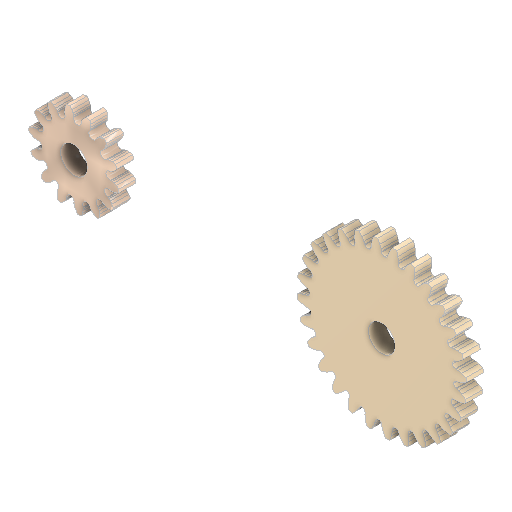
# Autodesk Inventor part: tool_kit
Saved by Autodesk Inventor 2025.3 (Build 293356030, 356C)
## iProperties
Created: 2025-09-03
Part Number: tool_kit
Material: 一般
Document SubType Name: Modeling
Designer: 陳泓任
Density: 1 g/cm^3
Appearance: 一般
Author: 陳泓任
Autodesk Inventor part; units mm, degrees
(part 1 of 2)
ref_plane "YZ Plane" through (0, 0, 0) normal (1, 0, 0) x (0, 1, 0)
ref_plane "XZ Plane" through (0, 0, 0) normal (0, 1, 0) x (-1, 0, 0)
ref_plane "XY Plane" through (0, 0, 0) normal (0, 0, 1) x (1, 0, 0)
sketch "草圖2" plane through (0, 0, 0) normal (0, 0, 1) x (1, 0, 0)
  circle A0 centre (1.2232, 0.0647) radius 2.34
  arc A1 (5.8477, -6.4632) -> (5.8053, -5.9159) centre (1.4586, -6.5279) ccw
  arc A2 (5.8053, -5.9159) -> (5.7115, -5.4774) centre (2.6173, -6.3691) ccw
  arc A3 (5.7115, -5.4774) -> (5.6019, -5.1764) centre (3.4971, -6.1133) ccw
  arc A4 (5.6019, -5.1764) -> (5.5121, -5.0064) centre (4.3299, -5.7392) ccw
  arc A5 (5.5121, -5.0064) -> (5.4754, -4.9539) centre (5.071, -5.2755) ccw
  line L0 (5.4754, -4.9539) -> (5.4708, -4.9484)
  arc A6 (6.3664, -4.0369) -> (5.4708, -4.9484) centre (5.8051, -4.3811) ccw
  arc A7 (6.3664, -4.0369) -> (6.4195, -4.0716) centre (6.6754, -3.6228) ccw
  arc A8 (6.4195, -4.0716) -> (6.5921, -4.1563) centre (7.1169, -2.8681) ccw
  arc A9 (6.5921, -4.1563) -> (6.8962, -4.2569) centre (7.466, -2.0246) ccw
  arc A10 (6.8962, -4.2569) -> (7.3374, -4.3377) centre (7.6956, -1.1376) ccw
  arc A11 (7.3374, -4.3377) -> (7.8856, -4.3638) centre (7.8199, 0.0253) ccw
  arc A12 (8.2221, -3.8102) -> (7.9465, -3.3355) centre (4.2957, -5.7729) ccw
  arc A13 (7.9465, -3.3355) -> (7.6716, -2.9812) centre (5.2708, -5.1271) ccw
  arc A14 (7.6716, -2.9812) -> (7.4423, -2.7575) centre (5.9524, -4.5148) ccw
  arc A15 (7.4423, -2.7575) -> (7.2877, -2.6433) centre (6.5404, -3.8165) ccw
  arc A16 (7.2877, -2.6433) -> (7.2318, -2.6119) centre (7.007, -3.0771) ccw
  line L1 (7.2318, -2.6119) -> (7.2252, -2.609)
  arc A17 (7.6367, -1.3991) -> (7.2252, -2.609) centre (7.2803, -1.9528) ccw
  arc A18 (7.6367, -1.3991) -> (7.6996, -1.4074) centre (7.7354, -0.8919) ccw
  arc A19 (7.6996, -1.4074) -> (7.8918, -1.4088) centre (7.8057, -0.0205) ccw
  arc A20 (7.8918, -1.4088) -> (8.2095, -1.3675) centre (7.7543, 0.891) ccw
  arc A21 (8.2095, -1.3675) -> (8.642, -1.2489) centre (7.5763, 1.7897) ccw
  arc A22 (8.642, -1.2489) -> (9.1473, -1.0345) centre (7.1837, 2.8914) ccw
  arc A23 (9.2102, -0.3897) -> (8.756, -0.0817) centre (6.5243, -3.8616) ccw
  arc A24 (8.756, -0.0817) -> (8.3546, 0.1183) centre (7.1226, -2.8567) ccw
  arc A25 (8.3546, 0.1183) -> (8.0509, 0.2203) centre (7.4711, -2.0094) ccw
  arc A26 (8.0509, 0.2203) -> (7.8621, 0.2562) centre (7.6979, -1.1251) ccw
  arc A27 (7.8621, 0.2562) -> (7.7981, 0.2602) centre (7.7974, -0.2565) ccw
  line L2 (7.7981, 0.2602) -> (7.7909, 0.26)
  arc A28 (7.6367, 1.5286) -> (7.7909, 0.26) centre (7.5559, 0.8751) ccw
  arc A29 (7.6367, 1.5286) -> (7.697, 1.5484) centre (7.5055, 2.0283) ccw
  arc A30 (7.697, 1.5484) -> (7.8707, 1.6306) centre (7.1908, 2.844) ccw
  arc A31 (7.8707, 1.6306) -> (8.139, 1.8056) centre (6.749, 3.6429) ccw
  arc A32 (8.139, 1.8056) -> (8.4772, 2.1001) centre (6.1987, 4.3754) ccw
  arc A33 (8.4772, 2.1001) -> (8.8395, 2.5125) centre (5.3669, 5.1976) ccw
  arc A34 (8.6164, 3.1207) -> (8.0735, 3.2012) centre (7.7029, -1.1727) ccw
  arc A35 (8.0735, 3.2012) -> (7.6251, 3.2072) centre (7.8059, -0.0077) ccw
  arc A36 (7.6251, 3.2072) -> (7.3072, 3.1674) centre (7.7522, 0.9069) ccw
  arc A37 (7.3072, 3.1674) -> (7.1215, 3.1177) centre (7.5729, 1.802) ccw
  arc A38 (7.1215, 3.1177) -> (7.0622, 3.0936) centre (7.2857, 2.6278) ccw
  line L3 (7.0622, 3.0936) -> (7.0558, 3.0903)
  arc A39 (6.3664, 4.1663) -> (7.0558, 3.0903) centre (6.5771, 3.5425) ccw
  arc A40 (6.3664, 4.1663) -> (6.4121, 4.2104) centre (6.0314, 4.5597) ccw
  arc A41 (6.4121, 4.2104) -> (6.533, 4.3598) centre (5.3939, 5.158) ccw
  arc A42 (6.533, 4.3598) -> (6.6988, 4.6339) centre (4.6492, 5.6861) ccw
  arc A43 (6.6988, 4.6339) -> (6.8757, 5.046) centre (3.8356, 6.1073) ccw
  arc A44 (6.8757, 5.046) -> (7.0232, 5.5747) centre (2.7295, 6.4872) ccw
  arc A45 (6.5583, 6.0259) -> (6.0342, 5.8628) centre (7.5981, 1.7613) ccw
  arc A46 (6.0342, 5.8628) -> (5.6276, 5.6737) centre (7.1855, 2.8556) ccw
  arc A47 (5.6276, 5.6737) -> (5.3585, 5.4999) centre (6.7402, 3.6563) ccw
  arc A48 (5.3585, 5.4999) -> (5.2128, 5.3746) centre (6.1903, 4.385) ccw
  arc A49 (5.2128, 5.3746) -> (5.1697, 5.3271) centre (5.5733, 5.0044) ccw
  line L4 (5.1697, 5.3271) -> (5.1654, 5.3214)
  arc A50 (4.0774, 5.9917) -> (5.1654, 5.3214) centre (4.538, 5.5211) ccw
  arc A51 (4.0774, 5.9917) -> (4.0995, 6.0512) centre (3.6049, 6.2008) ccw
  arc A52 (4.0995, 6.0512) -> (4.1436, 6.2383) centre (2.771, 6.4633) ccw
  arc A53 (4.1436, 6.2383) -> (4.174, 6.5572) centre (1.8709, 6.6159) ccw
  arc A54 (4.174, 6.5572) -> (4.1547, 7.0052) centre (0.9551, 6.6424) ccw
  arc A55 (4.1547, 7.0052) -> (4.0581, 7.5456) centre (-0.2063, 6.5048) ccw
  arc A56 (3.4435, 7.7504) -> (3.0421, 7.3761) centre (6.2307, 4.3592) ccw
  arc A57 (3.0421, 7.3761) -> (2.7578, 7.0293) centre (5.3841, 5.1662) ccw
  arc A58 (2.7578, 7.0293) -> (2.5908, 6.7559) centre (4.6355, 5.6944) ccw
  arc A59 (2.5908, 6.7559) -> (2.5138, 6.5798) centre (3.8239, 6.1123) ccw
  arc A60 (2.5138, 6.5798) -> (2.4956, 6.5183) centre (2.9992, 6.4027) ccw
  line L5 (2.4956, 6.5183) -> (2.4942, 6.5113)
  arc A61 (1.2231, 6.6432) -> (2.4942, 6.5113) centre (1.8423, 6.419) ccw
  arc A62 (1.2231, 6.6432) -> (1.2172, 6.7064) centre (0.7067, 6.6265) ccw
  arc A63 (1.2172, 6.7064) -> (1.1758, 6.8941) centre (-0.1585, 6.5012) ccw
  arc A64 (1.1758, 6.8941) -> (1.0648, 7.1946) centre (-1.0357, 6.2482) ccw
  arc A65 (1.0648, 7.1946) -> (0.853, 7.5898) centre (-1.8723, 5.8747) ccw
  arc A66 (0.853, 7.5898) -> (0.5315, 8.0348) centre (-2.859, 5.2468) ccw
  arc A67 (-0.1111, 7.9527) -> (-0.3103, 7.4412) centre (3.8715, 6.1066) ccw
  arc A68 (-0.3103, 7.4412) -> (-0.416, 7.0054) centre (2.7586, 6.4663) ccw
  arc A69 (-0.416, 7.0054) -> (-0.4479, 6.6866) centre (1.855, 6.6175) ccw
  arc A70 (-0.4479, 6.6866) -> (-0.4408, 6.4946) centre (0.9423, 6.6418) ccw
  arc A71 (-0.4408, 6.4946) -> (-0.4305, 6.4313) centre (0.0734, 6.5456) ccw
  line L6 (-0.4305, 6.4313) -> (-0.4287, 6.4244)
  arc A72 (-1.6311, 5.9917) -> (-0.4287, 6.4244) centre (-0.9761, 6.0583) ccw
  arc A73 (-1.6311, 5.9917) -> (-1.6639, 6.0461) centre (-2.0892, 5.7526) ccw
  arc A74 (-1.6639, 6.0461) -> (-1.7775, 6.1914) centre (-2.8144, 5.2643) ccw
  arc A75 (-1.7775, 6.1914) -> (-2.013, 6.4198) centre (-3.4949, 4.6558) ccw
  arc A76 (-2.013, 6.4198) -> (-2.3754, 6.684) centre (-4.0866, 3.9563) ccw
  arc A77 (-2.3754, 6.684) -> (-2.858, 6.9454) centre (-4.7032, 2.9624) ccw
  arc A78 (-3.4014, 6.5926) -> (-3.359, 6.0454) centre (0.9877, 6.6573) ccw
  arc A79 (-3.359, 6.0454) -> (-3.2651, 5.6068) centre (-0.171, 6.4986) ccw
  arc A80 (-3.2651, 5.6068) -> (-3.1555, 5.3058) centre (-1.0507, 6.2427) ccw
  arc A81 (-3.1555, 5.3058) -> (-3.0658, 5.1359) centre (-1.8836, 5.8686) ccw
  arc A82 (-3.0658, 5.1359) -> (-3.0291, 5.0833) centre (-2.6247, 5.4049) ccw
  line L7 (-3.0291, 5.0833) -> (-3.0245, 5.0778)
  arc A83 (-3.9201, 4.1663) -> (-3.0245, 5.0778) centre (-3.3588, 4.5106) ccw
  arc A84 (-3.9201, 4.1663) -> (-3.9732, 4.2011) centre (-4.2291, 3.7522) ccw
  arc A85 (-3.9732, 4.2011) -> (-4.1458, 4.2857) centre (-4.6705, 2.9976) ccw
  arc A86 (-4.1458, 4.2857) -> (-4.4499, 4.3863) centre (-5.0197, 2.154) ccw
  arc A87 (-4.4499, 4.3863) -> (-4.891, 4.4671) centre (-5.2493, 1.2671) ccw
  arc A88 (-4.891, 4.4671) -> (-5.4393, 4.4932) centre (-5.3735, 0.1041) ccw
  arc A89 (-5.7758, 3.9396) -> (-5.5002, 3.465) centre (-1.8494, 5.9023) ccw
  arc A90 (-5.5002, 3.465) -> (-5.2253, 3.1106) centre (-2.8245, 5.2565) ccw
  arc A91 (-5.2253, 3.1106) -> (-4.9959, 2.887) centre (-3.5061, 4.6443) ccw
  arc A92 (-4.9959, 2.887) -> (-4.8413, 2.7727) centre (-4.0941, 3.9459) ccw
  arc A93 (-4.8413, 2.7727) -> (-4.7855, 2.7413) centre (-4.5607, 3.2066) ccw
  line L8 (-4.7855, 2.7413) -> (-4.7789, 2.7384)
  arc A94 (-5.1904, 1.5285) -> (-4.7789, 2.7384) centre (-4.834, 2.0823) ccw
  arc A95 (-5.1904, 1.5285) -> (-5.2533, 1.5368) centre (-5.2891, 1.0214) ccw
  arc A96 (-5.2533, 1.5368) -> (-5.4455, 1.5382) centre (-5.3594, 0.1499) ccw
  arc A97 (-5.4455, 1.5382) -> (-5.7632, 1.4969) centre (-5.3079, -0.7616) ccw
  arc A98 (-5.7632, 1.4969) -> (-6.1957, 1.3783) centre (-5.13, -1.6603) ccw
  arc A99 (-6.1957, 1.3783) -> (-6.701, 1.1639) centre (-4.7374, -2.762) ccw
  arc A100 (-6.7522, 0.6928) -> (-6.7639, 0.5192) centre (1.2232, 0.0647) ccw
  arc A101 (-6.7639, 0.5192) -> (-6.3096, 0.2111) centre (-4.078, 3.9911) ccw
  arc A102 (-6.3096, 0.2111) -> (-5.9009, 0.0081) centre (-4.6763, 2.9861) ccw
  arc A103 (-5.9009, 0.0081) -> (-5.6046, -0.0909) centre (-5.0247, 2.1388) ccw
  arc A104 (-5.6046, -0.0909) -> (-5.4157, -0.1267) centre (-5.2515, 1.2545) ccw
  arc A105 (-5.4157, -0.1267) -> (-5.3518, -0.1308) centre (-5.3511, 0.3859) ccw
  line L9 (-5.3518, -0.1308) -> (-5.3446, -0.1306)
  arc A106 (-5.1903, -1.3991) -> (-5.3446, -0.1306) centre (-5.1095, -0.7457) ccw
  arc A107 (-5.1903, -1.3991) -> (-5.2506, -1.419) centre (-5.0592, -1.8989) ccw
  arc A108 (-5.2506, -1.419) -> (-5.4244, -1.5011) centre (-4.7445, -2.7146) ccw
  arc A109 (-5.4244, -1.5011) -> (-5.6927, -1.6762) centre (-4.3027, -3.5135) ccw
  arc A110 (-5.6927, -1.6762) -> (-6.0309, -1.9707) centre (-3.7524, -4.246) ccw
  arc A111 (-6.0309, -1.9707) -> (-6.3932, -2.3831) centre (-2.9206, -5.0682) ccw
  arc A112 (-6.1701, -2.9913) -> (-5.6272, -3.0718) centre (-5.2566, 1.3022) ccw
  arc A113 (-5.6272, -3.0718) -> (-5.1787, -3.0778) centre (-5.3596, 0.1372) ccw
  arc A114 (-5.1787, -3.0778) -> (-4.8609, -3.0379) centre (-5.3059, -0.7775) ccw
  arc A115 (-4.8609, -3.0379) -> (-4.6752, -2.9883) centre (-5.1266, -1.6726) ccw
  arc A116 (-4.6752, -2.9883) -> (-4.6158, -2.9642) centre (-4.8394, -2.4984) ccw
  line L10 (-4.6158, -2.9642) -> (-4.6095, -2.9609)
  arc A117 (-3.9201, -4.0369) -> (-4.6095, -2.9609) centre (-4.1308, -3.4131) ccw
  arc A118 (-3.9201, -4.0369) -> (-3.9658, -4.0809) centre (-3.5851, -4.4303) ccw
  arc A119 (-3.9658, -4.0809) -> (-4.0867, -4.2304) centre (-2.9476, -5.0286) ccw
  arc A120 (-4.0867, -4.2304) -> (-4.2488, -4.4974) centre (-2.2029, -5.5567) ccw
  arc A121 (-4.2488, -4.4974) -> (-4.4294, -4.9166) centre (-1.3893, -5.9779) ccw
  arc A122 (-4.4294, -4.9166) -> (-4.5769, -5.4453) centre (-0.2832, -6.3578) ccw
  arc A123 (-4.112, -5.8965) -> (-3.5879, -5.7334) centre (-5.1518, -1.6318) ccw
  arc A124 (-3.5879, -5.7334) -> (-3.1813, -5.5443) centre (-4.7392, -2.7262) ccw
  arc A125 (-3.1813, -5.5443) -> (-2.9122, -5.3705) centre (-4.2939, -3.5269) ccw
  arc A126 (-2.9122, -5.3705) -> (-2.7665, -5.2451) centre (-3.7439, -4.2556) ccw
  arc A127 (-2.7665, -5.2451) -> (-2.7234, -5.1977) centre (-3.1269, -4.875) ccw
  line L11 (-2.7234, -5.1977) -> (-2.7191, -5.1919)
  arc A128 (-1.6311, -5.8623) -> (-2.7191, -5.1919) centre (-2.0916, -5.3917) ccw
  arc A129 (-1.6311, -5.8623) -> (-1.6532, -5.9218) centre (-1.1586, -6.0713) ccw
  arc A130 (-1.6532, -5.9218) -> (-1.6973, -6.1089) centre (-0.3247, -6.3338) ccw
  arc A131 (-1.6973, -6.1089) -> (-1.7277, -6.4278) centre (0.5754, -6.4865) ccw
  arc A132 (-1.7277, -6.4278) -> (-1.7083, -6.8758) centre (1.4912, -6.513) ccw
  arc A133 (-1.7083, -6.8758) -> (-1.6118, -7.4161) centre (2.6526, -6.3754) ccw
  arc A134 (-0.9972, -7.621) -> (-0.5958, -7.2467) centre (-3.7844, -4.2298) ccw
  arc A135 (-0.5958, -7.2467) -> (-0.3114, -6.8998) centre (-2.9378, -5.0367) ccw
  arc A136 (-0.3114, -6.8998) -> (-0.1444, -6.6265) centre (-2.1892, -5.565) ccw
  arc A137 (-0.1444, -6.6265) -> (-0.0675, -6.4503) centre (-1.3775, -5.9829) ccw
  arc A138 (-0.0675, -6.4503) -> (-0.0493, -6.3889) centre (-0.5529, -6.2733) ccw
  line L12 (-0.0493, -6.3889) -> (-0.0479, -6.3818)
  arc A139 (1.2232, -6.5137) -> (-0.0479, -6.3818) centre (0.604, -6.2895) ccw
  arc A140 (1.2232, -6.5137) -> (1.2291, -6.5769) centre (1.7396, -6.4971) ccw
  arc A141 (1.2291, -6.5769) -> (1.2705, -6.7646) centre (2.6048, -6.3718) ccw
  arc A142 (1.2705, -6.7646) -> (1.3815, -7.0651) centre (3.482, -6.1188) ccw
  arc A143 (1.3815, -7.0651) -> (1.5934, -7.4604) centre (4.3186, -5.7453) ccw
  arc A144 (1.5934, -7.4604) -> (1.9148, -7.9053) centre (5.3053, -5.1174) ccw
  arc A145 (2.5574, -7.8232) -> (2.7567, -7.3118) centre (-1.4251, -5.9772) ccw
  arc A146 (2.7567, -7.3118) -> (2.8623, -6.876) centre (-0.3123, -6.3369) ccw
  arc A147 (2.8623, -6.876) -> (2.8944, -6.5495) centre (0.5914, -6.4881) ccw
  arc A148 (2.8944, -6.5495) -> (2.8871, -6.3651) centre (1.504, -6.5124) ccw
  arc A149 (2.8871, -6.3651) -> (2.8768, -6.3019) centre (2.3729, -6.4162) ccw
  line L13 (2.8768, -6.3019) -> (2.875, -6.2949)
  arc A150 (4.0775, -5.8623) -> (2.875, -6.2949) centre (3.4224, -5.9289) ccw
  arc A151 (4.0775, -5.8623) -> (4.1102, -5.9166) centre (4.5355, -5.6232) ccw
  arc A152 (4.1102, -5.9166) -> (4.2238, -6.062) centre (5.2607, -5.1349) ccw
  arc A153 (4.2238, -6.062) -> (4.4593, -6.2904) centre (5.9412, -4.5263) ccw
  arc A154 (4.4593, -6.2904) -> (4.8217, -6.5546) centre (6.533, -3.8269) ccw
  arc A155 (4.8217, -6.5546) -> (5.3044, -6.816) centre (7.1495, -2.833) ccw
  circle A156 centre (55.7173, -0.0187) radius 2.34
  arc A157 (58.5817, 13.954) -> (58.37, 14.7449) centre (52.2673, 12.6876) ccw
  arc A158 (58.6643, 13.3186) -> (58.5817, 13.954) centre (54.0648, 13.0435) ccw
  arc A159 (58.6615, 12.9342) -> (58.6643, 13.3186) centre (55.8878, 13.1464) ccw
  arc A160 (58.6513, 12.844) -> (58.6615, 12.9342) centre (57.6307, 13.0057) ccw
  arc A161 (58.6513, 12.844) -> (59.051, 12.288) centre (59.177, 12.8002) ccw
  line L14 (59.051, 12.288) -> (59.0514, 12.2894)
  arc A162 (59.0514, 12.2894) -> (59.0647, 12.2848) centre (59.2291, 12.7861) ccw
  arc A163 (59.0647, 12.2848) -> (59.0785, 12.282) centre (59.177, 12.8002) ccw
  line L15 (59.0785, 12.282) -> (59.0782, 12.2806)
  arc A164 (59.0782, 12.2806) -> (59.7045, 12.5575) centre (59.2291, 12.7861) ccw
  arc A165 (59.7413, 12.6404) -> (59.7045, 12.5575) centre (60.6663, 12.1798) ccw
  arc A166 (59.9337, 12.9733) -> (59.7413, 12.6404) centre (62.2403, 11.4181) ccw
  arc A167 (60.3268, 13.4792) -> (59.9337, 12.9733) centre (63.7598, 10.4058) ccw
  arc A168 (60.91, 14.0538) -> (60.3268, 13.4792) centre (65.1293, 9.1883) ccw
  arc A169 (61.6191, 12.9663) -> (61.5887, 13.7845) centre (55.1812, 13.1367) ccw
  arc A170 (61.5583, 12.3285) -> (61.6191, 12.9663) centre (57.0128, 13.0837) ccw
  arc A171 (61.47, 11.9543) -> (61.5583, 12.3285) centre (58.813, 12.7784) ccw
  arc A172 (61.44, 11.8687) -> (61.47, 11.9543) centre (60.4809, 12.2534) ccw
  arc A173 (61.44, 11.8687) -> (61.7059, 11.2376) centre (61.9427, 11.709) ccw
  line L16 (61.7059, 11.2376) -> (61.7066, 11.2389)
  arc A174 (61.7066, 11.2389) -> (61.7186, 11.2315) centre (61.9903, 11.6836) ccw
  arc A175 (61.7186, 11.2315) -> (61.7314, 11.2257) centre (61.9427, 11.709) ccw
  line L17 (61.7314, 11.2257) -> (61.7308, 11.2244)
  arc A176 (61.7308, 11.2244) -> (62.403, 11.355) centre (61.9903, 11.6836) ccw
  arc A177 (62.4574, 11.4276) -> (62.403, 11.355) centre (63.2567, 10.7727) ccw
  arc A178 (62.719, 11.7093) -> (62.4574, 11.4276) centre (64.6216, 9.6799) ccw
  arc A179 (63.2148, 12.115) -> (62.719, 11.7093) centre (65.8779, 8.3548) ccw
  arc A180 (63.9113, 12.5455) -> (63.2148, 12.115) centre (66.942, 6.8631) ccw
  arc A181 (64.3605, 11.3274) -> (64.513, 12.1319) centre (58.122, 12.9262) ccw
  arc A182 (64.1593, 10.7192) -> (64.3605, 11.3274) centre (59.8959, 12.467) ccw
  arc A183 (63.99, 10.374) -> (64.1593, 10.7192) centre (61.583, 11.7687) ccw
  arc A184 (63.9417, 10.2972) -> (63.99, 10.374) centre (63.0923, 10.8857) ccw
  arc A185 (63.9417, 10.2972) -> (64.0605, 9.6228) centre (64.3963, 10.0297) ccw
  line L18 (64.0605, 9.6228) -> (64.0615, 9.6239)
  arc A186 (64.0615, 9.6239) -> (64.0715, 9.614) centre (64.4371, 9.9943) ccw
  arc A187 (64.0715, 9.614) -> (64.0828, 9.6055) centre (64.3963, 10.0297) ccw
  line L19 (64.0828, 9.6055) -> (64.0818, 9.6044)
  arc A188 (64.0818, 9.6044) -> (64.7662, 9.5821) centre (64.4371, 9.9943) ccw
  arc A189 (64.8354, 9.6409) -> (64.7662, 9.5821) centre (65.469, 8.8245) ccw
  arc A190 (65.1531, 9.8572) -> (64.8354, 9.6409) centre (66.5565, 7.4553) ccw
  arc A191 (65.7268, 10.1425) -> (65.1531, 9.8572) centre (67.4864, 5.8839) ccw
  arc A192 (66.5016, 10.4072) -> (65.7268, 10.1425) centre (68.1919, 4.1928) ccw
  arc A193 (66.6686, 9.1197) -> (66.9962, 9.87) centre (60.9422, 12.0665) ccw
  arc A194 (66.3371, 8.5714) -> (66.6686, 9.1197) centre (62.5695, 11.2241) ccw
  arc A195 (66.0952, 8.2726) -> (66.3371, 8.5714) centre (64.0589, 10.1679) ccw
  arc A196 (66.031, 8.2085) -> (66.0952, 8.2726) centre (65.3338, 8.9713) ccw
  arc A197 (66.031, 8.2085) -> (65.9968, 7.5246) centre (66.4147, 7.8465) ccw
  line L20 (65.9968, 7.5246) -> (65.998, 7.5254)
  arc A198 (65.998, 7.5254) -> (66.0055, 7.5135) centre (66.4466, 7.8029) ccw
  arc A199 (66.0055, 7.5135) -> (66.0146, 7.5027) centre (66.4147, 7.8465) ccw
  line L21 (66.0146, 7.5027) -> (66.0134, 7.5018)
  arc A200 (66.0134, 7.5018) -> (66.6758, 7.3278) centre (66.4466, 7.8029) ccw
  arc A201 (66.7563, 7.3697) -> (66.6758, 7.3278) centre (67.1923, 6.4328) ccw
  arc A202 (67.1142, 7.51) -> (66.7563, 7.3697) centre (67.9479, 4.856) ccw
  arc A203 (67.7369, 7.6604) -> (67.1142, 7.51) centre (68.5048, 3.1171) ccw
  arc A204 (68.5512, 7.746) -> (67.7369, 7.6604) centre (68.8163, 1.3114) ccw
  arc A205 (68.4275, 6.4537) -> (68.9139, 7.1123) centre (63.5005, 10.6009) ccw
  arc A206 (67.9823, 5.993) -> (68.4275, 6.4537) centre (64.8994, 9.4175) ccw
  arc A207 (67.68, 5.7554) -> (67.9823, 5.993) centre (66.1165, 8.0563) ccw
  arc A208 (67.6031, 5.7072) -> (67.68, 5.7554) centre (67.0932, 6.606) ccw
  arc A209 (67.6031, 5.7072) -> (67.4176, 5.0481) centre (67.8966, 5.2689) ccw
  line L22 (67.4176, 5.0481) -> (67.4189, 5.0486)
  arc A210 (67.4189, 5.0486) -> (67.4237, 5.0353) centre (67.918, 5.2194) ccw
  arc A211 (67.4237, 5.0353) -> (67.4301, 5.0228) centre (67.8966, 5.2689) ccw
  line L23 (67.4301, 5.0228) -> (67.4288, 5.0222)
  arc A212 (67.4288, 5.0222) -> (68.0358, 4.7052) centre (67.918, 5.2194) ccw
  arc A213 (68.1236, 4.7281) -> (68.0358, 4.7052) centre (68.3402, 3.7177) ccw
  arc A214 (68.5037, 4.7852) -> (68.1236, 4.7281) centre (68.726, 2.0122) ccw
  arc A215 (69.1443, 4.7933) -> (68.5037, 4.7852) centre (68.882, 0.193) ccw
  arc A216 (69.9573, 4.6956) -> (69.1443, 4.7933) centre (68.7839, -1.6368) ccw
  arc A217 (69.5491, 3.4631) -> (70.1698, 3.997) centre (65.6684, 8.6027) ccw
  arc A218 (69.0125, 3.113) -> (69.5491, 3.4631) centre (66.769, 7.1377) ccw
  arc A219 (68.665, 2.9487) -> (69.0125, 3.113) centre (67.6526, 5.5399) ccw
  arc A220 (68.5793, 2.9188) -> (68.665, 2.9487) centre (68.2821, 3.9085) ccw
  arc A221 (68.5793, 2.9188) -> (68.2517, 2.3175) centre (68.7679, 2.4262) ccw
  line L24 (68.2517, 2.3175) -> (68.2531, 2.3177)
  arc A222 (68.2531, 2.3177) -> (68.2548, 2.3037) centre (68.7777, 2.3731) ccw
  arc A223 (68.2548, 2.3037) -> (68.2583, 2.29) centre (68.7679, 2.4262) ccw
  line L25 (68.2583, 2.29) -> (68.2568, 2.2898)
  arc A224 (68.2568, 2.2898) -> (68.7781, 1.8456) centre (68.7777, 2.3731) ccw
  arc A225 (68.8688, 1.8484) -> (68.7781, 1.8456) centre (68.8551, 0.8151) ccw
  arc A226 (69.2521, 1.8195) -> (68.8688, 1.8484) centre (68.8517, -0.9334) ccw
  arc A227 (69.8785, 1.6848) -> (69.2521, 1.8195) centre (68.599, -2.7417) ccw
  arc A228 (70.6493, 1.4087) -> (69.8785, 1.6848) centre (68.0962, -4.5038) ccw
  arc A229 (69.977, 0.298) -> (70.701, 0.6804) centre (67.3374, 6.1723) ccw
  arc A230 (69.376, 0.076) -> (69.977, 0.298) centre (68.0843, 4.499) ccw
  arc A231 (69.0006, -0.0068) -> (69.376, 0.076) centre (68.5903, 2.7446) ccw
  arc A232 (68.9105, -0.0169) -> (69.0006, -0.0068) centre (68.841, 1.0141) ccw
  arc A233 (68.9105, -0.0169) -> (68.4573, -0.5303) centre (68.9847, -0.5391) ccw
  line L26 (68.4573, -0.5303) -> (68.4587, -0.5303)
  arc A234 (68.4587, -0.5303) -> (68.4573, -0.5444) centre (68.9825, -0.5931) ccw
  arc A235 (68.4573, -0.5444) -> (68.4576, -0.5585) centre (68.9847, -0.5391) ccw
  line L27 (68.4576, -0.5585) -> (68.4561, -0.5584)
  arc A236 (68.4561, -0.5584) -> (68.8655, -1.1074) centre (68.9825, -0.5931) ccw
  arc A237 (68.9545, -1.1249) -> (68.8655, -1.1074) centre (68.7113, -2.1292) ccw
  arc A238 (69.3218, -1.2384) -> (68.9545, -1.1249) centre (68.3189, -3.8331) ccw
  arc A239 (69.9025, -1.509) -> (69.3218, -1.2384) centre (67.6701, -5.5399) ccw
  arc A240 (70.5925, -1.9498) -> (69.9025, -1.509) centre (66.7878, -7.1459) ccw
  arc A241 (69.69, -2.883) -> (70.4809, -2.6713) centre (68.4236, 3.4313) ccw
  arc A242 (69.0547, -2.9657) -> (69.69, -2.883) centre (68.7795, 1.6339) ccw
  arc A243 (68.6703, -2.9629) -> (69.0547, -2.9657) centre (68.8824, -0.1891) ccw
  arc A244 (68.5801, -2.9527) -> (68.6703, -2.9629) centre (68.7418, -1.932) ccw
  arc A245 (68.5801, -2.9527) -> (68.0241, -3.3524) centre (68.5363, -3.4783) ccw
  line L28 (68.0241, -3.3524) -> (68.0254, -3.3527)
  arc A246 (68.0254, -3.3527) -> (68.0209, -3.3661) centre (68.5221, -3.5304) ccw
  arc A247 (68.0209, -3.3661) -> (68.018, -3.3799) centre (68.5363, -3.4783) ccw
  line L29 (68.018, -3.3799) -> (68.0167, -3.3795)
  arc A248 (68.0167, -3.3795) -> (68.2936, -4.0058) centre (68.5221, -3.5304) ccw
  arc A249 (68.3765, -4.0427) -> (68.2936, -4.0058) centre (67.9159, -4.9677) ccw
  arc A250 (68.7093, -4.2351) -> (68.3765, -4.0427) centre (67.1542, -6.5416) ccw
  arc A251 (69.2152, -4.6282) -> (68.7093, -4.2351) centre (66.1418, -8.0612) ccw
  arc A252 (69.7899, -5.2114) -> (69.2152, -4.6282) centre (64.9243, -9.4306) ccw
  arc A253 (68.7023, -5.9204) -> (69.5205, -5.89) centre (68.8728, 0.5174) ccw
  arc A254 (68.0645, -5.8596) -> (68.7023, -5.9204) centre (68.8198, -1.3142) ccw
  arc A255 (67.6904, -5.7714) -> (68.0645, -5.8596) centre (68.5144, -3.1144) ccw
  arc A256 (67.6047, -5.7413) -> (67.6904, -5.7714) centre (67.9895, -4.7823) ccw
  arc A257 (67.6047, -5.7413) -> (66.9737, -6.0073) centre (67.445, -6.2441) ccw
  line L30 (66.9737, -6.0073) -> (66.975, -6.0079)
  arc A258 (66.975, -6.0079) -> (66.9675, -6.02) centre (67.4196, -6.2917) ccw
  arc A259 (66.9675, -6.02) -> (66.9617, -6.0328) centre (67.445, -6.2441) ccw
  line L31 (66.9617, -6.0328) -> (66.9604, -6.0321)
  arc A260 (66.9604, -6.0321) -> (67.091, -6.7044) centre (67.4196, -6.2917) ccw
  arc A261 (67.1637, -6.7587) -> (67.091, -6.7044) centre (66.5088, -7.558) ccw
  arc A262 (67.4453, -7.0203) -> (67.1637, -6.7587) centre (65.4159, -8.923) ccw
  arc A263 (67.8511, -7.5162) -> (67.4453, -7.0203) centre (64.0909, -10.1792) ccw
  arc A264 (68.2815, -8.2126) -> (67.8511, -7.5162) centre (62.5992, -11.2434) ccw
  arc A265 (67.0635, -8.6619) -> (67.8679, -8.8143) centre (68.6622, -2.4234) ccw
  arc A266 (66.4552, -8.4607) -> (67.0635, -8.6619) centre (68.203, -4.1973) ccw
  arc A267 (66.1101, -8.2914) -> (66.4552, -8.4607) centre (67.5047, -5.8844) ccw
  arc A268 (66.0333, -8.243) -> (66.1101, -8.2914) centre (66.6218, -7.3936) ccw
  arc A269 (66.0333, -8.243) -> (65.3589, -8.3619) centre (65.7657, -8.6977) ccw
  line L32 (65.3589, -8.3619) -> (65.36, -8.3628)
  arc A270 (65.36, -8.3628) -> (65.3501, -8.3729) centre (65.7304, -8.7384) ccw
  arc A271 (65.3501, -8.3729) -> (65.3415, -8.3841) centre (65.7657, -8.6977) ccw
  line L33 (65.3415, -8.3841) -> (65.3404, -8.3832)
  arc A272 (65.3404, -8.3832) -> (65.3182, -9.0676) centre (65.7304, -8.7384) ccw
  arc A273 (65.3769, -9.1368) -> (65.3182, -9.0676) centre (64.5605, -9.7703) ccw
  arc A274 (65.5933, -9.4545) -> (65.3769, -9.1368) centre (63.1914, -10.8579) ccw
  arc A275 (65.8785, -10.0282) -> (65.5933, -9.4545) centre (61.62, -11.7878) ccw
  arc A276 (66.1432, -10.803) -> (65.8785, -10.0282) centre (59.9289, -12.4933) ccw
  arc A277 (64.8557, -10.9699) -> (65.6061, -11.2976) centre (67.8026, -5.2436) ccw
  arc A278 (64.3075, -10.6384) -> (64.8557, -10.9699) centre (66.9601, -6.8708) ccw
  arc A279 (64.0087, -10.3966) -> (64.3075, -10.6384) centre (65.904, -8.3603) ccw
  arc A280 (63.9446, -10.3324) -> (64.0087, -10.3966) centre (64.7073, -9.6352) ccw
  arc A281 (63.9446, -10.3324) -> (63.2606, -10.2982) centre (63.5826, -10.716) ccw
  line L34 (63.2606, -10.2982) -> (63.2615, -10.2993)
  arc A282 (63.2615, -10.2993) -> (63.2496, -10.3069) centre (63.539, -10.7479) ccw
  arc A283 (63.2496, -10.3069) -> (63.2387, -10.316) centre (63.5826, -10.716) ccw
  line L35 (63.2387, -10.316) -> (63.2379, -10.3148)
  arc A284 (63.2379, -10.3148) -> (63.0639, -10.9771) centre (63.539, -10.7479) ccw
  arc A285 (63.1057, -11.0576) -> (63.0639, -10.9771) centre (62.1689, -11.4936) ccw
  arc A286 (63.246, -11.4155) -> (63.1057, -11.0576) centre (60.592, -12.2493) ccw
  arc A287 (63.3964, -12.0383) -> (63.246, -11.4155) centre (58.8531, -12.8062) ccw
  arc A288 (63.4821, -12.8526) -> (63.3964, -12.0383) centre (57.0474, -13.1177) ccw
  arc A289 (62.1897, -12.7289) -> (62.8484, -13.2152) centre (66.3369, -7.8018) ccw
  arc A290 (61.729, -12.2837) -> (62.1897, -12.7289) centre (65.1535, -9.2008) ccw
  arc A291 (61.4915, -11.9814) -> (61.729, -12.2837) centre (63.7924, -10.4179) ccw
  arc A292 (61.4433, -11.9045) -> (61.4915, -11.9814) centre (62.342, -11.3946) ccw
  arc A293 (61.4433, -11.9045) -> (60.7841, -11.719) centre (61.005, -12.198) ccw
  line L36 (60.7841, -11.719) -> (60.7847, -11.7203)
  arc A294 (60.7847, -11.7203) -> (60.7714, -11.725) centre (60.9554, -12.2194) ccw
  arc A295 (60.7714, -11.725) -> (60.7588, -11.7315) centre (61.005, -12.198) ccw
  line L37 (60.7588, -11.7315) -> (60.7582, -11.7301)
  arc A296 (60.7582, -11.7301) -> (60.4412, -12.3371) centre (60.9554, -12.2194) ccw
  arc A297 (60.4641, -12.4249) -> (60.4412, -12.3371) centre (59.4537, -12.6415) ccw
  arc A298 (60.5212, -12.8051) -> (60.4641, -12.4249) centre (57.7483, -13.0273) ccw
  arc A299 (60.5293, -13.4457) -> (60.5212, -12.8051) centre (55.929, -13.1833) ccw
  arc A300 (60.4316, -14.2586) -> (60.5293, -13.4457) centre (54.0993, -13.0853) ccw
  arc A301 (59.1992, -13.8504) -> (59.7331, -14.4712) centre (64.3388, -9.9698) ccw
  arc A302 (58.8491, -13.3139) -> (59.1992, -13.8504) centre (62.8737, -11.0703) ccw
  arc A303 (58.6848, -12.9663) -> (58.8491, -13.3139) centre (61.2759, -11.954) ccw
  arc A304 (58.6549, -12.8806) -> (58.6848, -12.9663) centre (59.6446, -12.5835) ccw
  arc A305 (58.6549, -12.8806) -> (58.0535, -12.5531) centre (58.1623, -13.0693) ccw
  line L38 (58.0535, -12.5531) -> (58.0538, -12.5545)
  arc A306 (58.0538, -12.5545) -> (58.0398, -12.5562) centre (58.1092, -13.0791) ccw
  arc A307 (58.0398, -12.5562) -> (58.0261, -12.5596) centre (58.1623, -13.0693) ccw
  line L39 (58.0261, -12.5596) -> (58.0258, -12.5582)
  arc A308 (58.0258, -12.5582) -> (57.5817, -13.0794) centre (58.1092, -13.0791) ccw
  arc A309 (57.5844, -13.1701) -> (57.5817, -13.0794) centre (56.5512, -13.1565) ccw
  arc A310 (57.5555, -13.5535) -> (57.5844, -13.1701) centre (54.8026, -13.1531) ccw
  arc A311 (57.4209, -14.1798) -> (57.5555, -13.5535) centre (52.9943, -12.9004) ccw
  arc A312 (57.1447, -14.9506) -> (57.4209, -14.1798) centre (51.2323, -12.3976) ccw
  arc A313 (56.034, -14.2784) -> (56.4164, -15.0024) centre (61.9083, -11.6387) ccw
  arc A314 (55.8121, -13.6774) -> (56.034, -14.2784) centre (60.2351, -12.3857) ccw
  arc A315 (55.7293, -13.302) -> (55.8121, -13.6774) centre (58.4807, -12.8917) ccw
  arc A316 (55.7192, -13.2118) -> (55.7293, -13.302) centre (56.7502, -13.1423) ccw
  arc A317 (55.7192, -13.2118) -> (55.2058, -12.7587) centre (55.1969, -13.2861) ccw
  line L40 (55.2058, -12.7587) -> (55.2057, -12.7601)
  arc A318 (55.2057, -12.7601) -> (55.1917, -12.7586) centre (55.143, -13.2839) ccw
  arc A319 (55.1917, -12.7586) -> (55.1776, -12.759) centre (55.1969, -13.2861) ccw
  line L41 (55.1776, -12.759) -> (55.1776, -12.7575)
  arc A320 (55.1776, -12.7575) -> (54.6286, -13.1668) centre (55.143, -13.2839) ccw
  arc A321 (54.6112, -13.2559) -> (54.6286, -13.1668) centre (53.6069, -13.0126) ccw
  arc A322 (54.4977, -13.6232) -> (54.6112, -13.2559) centre (51.9029, -12.6203) ccw
  arc A323 (54.227, -14.2039) -> (54.4977, -13.6232) centre (50.1961, -11.9715) ccw
  arc A324 (53.7863, -14.8939) -> (54.227, -14.2039) centre (48.5902, -11.0892) ccw
  arc A325 (52.853, -13.9914) -> (53.0647, -14.7823) centre (59.1674, -12.725) ccw
  arc A326 (52.7704, -13.356) -> (52.853, -13.9914) centre (57.3699, -13.0809) ccw
  arc A327 (52.7731, -12.9716) -> (52.7704, -13.356) centre (55.5469, -13.1838) ccw
  arc A328 (52.7834, -12.8815) -> (52.7731, -12.9716) centre (53.804, -13.0431) ccw
  arc A329 (52.7834, -12.8815) -> (52.3837, -12.3254) centre (52.2577, -12.8377) ccw
  line L42 (52.3837, -12.3254) -> (52.3833, -12.3268)
  arc A330 (52.3833, -12.3268) -> (52.37, -12.3222) centre (52.2056, -12.8235) ccw
  arc A331 (52.37, -12.3222) -> (52.3561, -12.3194) centre (52.2577, -12.8377) ccw
  line L43 (52.3561, -12.3194) -> (52.3565, -12.318)
  arc A332 (52.3565, -12.318) -> (51.7302, -12.5949) centre (52.2056, -12.8235) ccw
  arc A333 (51.6934, -12.6779) -> (51.7302, -12.5949) centre (50.7683, -12.2172) ccw
  arc A334 (51.501, -13.0107) -> (51.6934, -12.6779) centre (49.1944, -11.4555) ccw
  arc A335 (51.1079, -13.5166) -> (51.501, -13.0107) centre (47.6748, -10.4432) ccw
  arc A336 (50.5246, -14.0912) -> (51.1079, -13.5166) centre (46.3054, -9.2257) ccw
  arc A337 (49.8156, -13.0037) -> (49.846, -13.8219) centre (56.2535, -13.1741) ccw
  arc A338 (49.8764, -12.3659) -> (49.8156, -13.0037) centre (54.4218, -13.1211) ccw
  arc A339 (49.9647, -11.9917) -> (49.8764, -12.3659) centre (52.6217, -12.8158) ccw
  arc A340 (49.9947, -11.9061) -> (49.9647, -11.9917) centre (50.9538, -12.2908) ccw
  arc A341 (49.9947, -11.9061) -> (49.7288, -11.2751) centre (49.492, -11.7464) ccw
  line L44 (49.7288, -11.2751) -> (49.7281, -11.2763)
  arc A342 (49.7281, -11.2763) -> (49.7161, -11.2689) centre (49.4443, -11.721) ccw
  arc A343 (49.7161, -11.2689) -> (49.7032, -11.2631) centre (49.492, -11.7464) ccw
  line L45 (49.7032, -11.2631) -> (49.7039, -11.2618)
  arc A344 (49.7039, -11.2618) -> (49.0317, -11.3924) centre (49.4443, -11.721) ccw
  arc A345 (48.9773, -11.465) -> (49.0317, -11.3924) centre (48.178, -10.8101) ccw
  arc A346 (48.7157, -11.7467) -> (48.9773, -11.465) centre (46.813, -9.7173) ccw
  arc A347 (48.2199, -12.1524) -> (48.7157, -11.7467) centre (45.5568, -8.3922) ccw
  arc A348 (47.5234, -12.5829) -> (48.2199, -12.1524) centre (44.4926, -6.9005) ccw
  arc A349 (47.0741, -11.3648) -> (46.9217, -12.1693) centre (53.3127, -12.9636) ccw
  arc A350 (47.2754, -10.7566) -> (47.0741, -11.3648) centre (51.5388, -12.5044) ccw
  arc A351 (47.4446, -10.4114) -> (47.2754, -10.7566) centre (49.8516, -11.8061) ccw
  arc A352 (47.493, -10.3347) -> (47.4446, -10.4114) centre (48.3424, -10.9231) ccw
  arc A353 (47.493, -10.3347) -> (47.3741, -9.6603) centre (47.0384, -10.0671) ccw
  line L46 (47.3741, -9.6603) -> (47.3732, -9.6613)
  arc A354 (47.3732, -9.6613) -> (47.3632, -9.6514) centre (46.9976, -10.0317) ccw
  arc A355 (47.3632, -9.6514) -> (47.3519, -9.6429) centre (47.0384, -10.0671) ccw
  line L47 (47.3519, -9.6429) -> (47.3529, -9.6418)
  arc A356 (47.3529, -9.6418) -> (46.6684, -9.6195) centre (46.9976, -10.0317) ccw
  arc A357 (46.5993, -9.6783) -> (46.6684, -9.6195) centre (45.9657, -8.8619) ccw
  arc A358 (46.2815, -9.8947) -> (46.5993, -9.6783) centre (44.8781, -7.4927) ccw
  arc A359 (45.7078, -10.1799) -> (46.2815, -9.8947) centre (43.9483, -5.9213) ccw
  arc A360 (44.933, -10.4446) -> (45.7078, -10.1799) centre (43.2427, -4.2302) ccw
  arc A361 (44.7661, -9.1571) -> (44.4385, -9.9074) centre (50.4924, -12.104) ccw
  arc A362 (45.0976, -8.6088) -> (44.7661, -9.1571) centre (48.8652, -11.2615) ccw
  arc A363 (45.3395, -8.31) -> (45.0976, -8.6088) centre (47.3758, -10.2053) ccw
  arc A364 (45.4037, -8.2459) -> (45.3395, -8.31) centre (46.1008, -9.0087) ccw
  arc A365 (45.4037, -8.2459) -> (45.4379, -7.562) centre (45.02, -7.8839) ccw
  line L48 (45.4379, -7.562) -> (45.4367, -7.5628)
  arc A366 (45.4367, -7.5628) -> (45.4291, -7.5509) centre (44.9881, -7.8404) ccw
  arc A367 (45.4291, -7.5509) -> (45.4201, -7.5401) centre (45.02, -7.8839) ccw
  line L49 (45.4201, -7.5401) -> (45.4212, -7.5393)
  arc A368 (45.4212, -7.5393) -> (44.7589, -7.3652) centre (44.9881, -7.8404) ccw
  arc A369 (44.6784, -7.4071) -> (44.7589, -7.3652) centre (44.2424, -6.4702) ccw
  arc A370 (44.3205, -7.5474) -> (44.6784, -7.4071) centre (43.4868, -4.8934) ccw
  arc A371 (43.6977, -7.6978) -> (44.3205, -7.5474) centre (42.9299, -3.1545) ccw
  arc A372 (42.8834, -7.7834) -> (43.6977, -7.6978) centre (42.6183, -1.3488) ccw
  arc A373 (43.0072, -6.4911) -> (42.5208, -7.1497) centre (47.9342, -10.6383) ccw
  arc A374 (43.4524, -6.0304) -> (43.0072, -6.4911) centre (46.5352, -9.4549) ccw
  arc A375 (43.7547, -5.7929) -> (43.4524, -6.0304) centre (45.3182, -8.0938) ccw
  arc A376 (43.8315, -5.7446) -> (43.7547, -5.7929) centre (44.3415, -6.6434) ccw
  arc A377 (43.8315, -5.7446) -> (44.0171, -5.0855) centre (43.538, -5.3063) ccw
  line L50 (44.0171, -5.0855) -> (44.0157, -5.086)
  arc A378 (44.0157, -5.086) -> (44.011, -5.0727) centre (43.5166, -5.2568) ccw
  arc A379 (44.011, -5.0727) -> (44.0046, -5.0602) centre (43.538, -5.3063) ccw
  line L51 (44.0046, -5.0602) -> (44.0059, -5.0596)
  arc A380 (44.0059, -5.0596) -> (43.3989, -4.7426) centre (43.5166, -5.2568) ccw
  arc A381 (43.3111, -4.7655) -> (43.3989, -4.7426) centre (43.0945, -3.7551) ccw
  arc A382 (42.931, -4.8226) -> (43.3111, -4.7655) centre (42.7087, -2.0496) ccw
  arc A383 (42.2903, -4.8307) -> (42.931, -4.8226) centre (42.5527, -0.2304) ccw
  arc A384 (41.4774, -4.733) -> (42.2903, -4.8307) centre (42.6508, 1.5994) ccw
  arc A385 (41.8856, -3.5005) -> (41.2649, -4.0344) centre (45.7663, -8.6401) ccw
  arc A386 (42.4222, -3.1504) -> (41.8856, -3.5005) centre (44.6657, -7.1751) ccw
  arc A387 (42.7697, -2.9861) -> (42.4222, -3.1504) centre (43.782, -5.5773) ccw
  arc A388 (42.8554, -2.9562) -> (42.7697, -2.9861) centre (43.1526, -3.9459) ccw
  arc A389 (42.8554, -2.9562) -> (43.183, -2.3549) centre (42.6668, -2.4636) ccw
  line L52 (43.183, -2.3549) -> (43.1815, -2.3551)
  arc A390 (43.1815, -2.3551) -> (43.1799, -2.3411) centre (42.657, -2.4105) ccw
  arc A391 (43.1799, -2.3411) -> (43.1764, -2.3274) centre (42.6668, -2.4636) ccw
  line L53 (43.1764, -2.3274) -> (43.1778, -2.3272)
  arc A392 (43.1778, -2.3272) -> (42.6566, -1.883) centre (42.657, -2.4105) ccw
  arc A393 (42.5659, -1.8858) -> (42.6566, -1.883) centre (42.5796, -0.8526) ccw
  arc A394 (42.1826, -1.8569) -> (42.5659, -1.8858) centre (42.5829, 0.896) ccw
  arc A395 (41.5562, -1.7222) -> (42.1826, -1.8569) centre (42.8357, 2.7043) ccw
  arc A396 (40.7854, -1.4461) -> (41.5562, -1.7222) centre (43.3384, 4.4664) ccw
  arc A397 (41.4576, -0.3354) -> (40.7336, -0.7178) centre (44.0973, -6.2097) ccw
  arc A398 (42.0586, -0.1135) -> (41.4576, -0.3354) centre (43.3504, -4.5364) ccw
  arc A399 (42.434, -0.0306) -> (42.0586, -0.1135) centre (42.8444, -2.782) ccw
  arc A400 (42.5242, -0.0205) -> (42.434, -0.0306) centre (42.5937, -1.0516) ccw
  arc A401 (42.5242, -0.0205) -> (42.9774, 0.4929) centre (42.4499, 0.5017) ccw
  line L54 (42.9774, 0.4929) -> (42.9759, 0.4929)
  arc A402 (42.9759, 0.4929) -> (42.9774, 0.507) centre (42.4522, 0.5556) ccw
  arc A403 (42.9774, 0.507) -> (42.9771, 0.5211) centre (42.4499, 0.5017) ccw
  line L55 (42.9771, 0.5211) -> (42.9785, 0.521)
  arc A404 (42.9785, 0.521) -> (42.5692, 1.07) centre (42.4522, 0.5556) ccw
  arc A405 (42.4802, 1.0875) -> (42.5692, 1.07) centre (42.7234, 2.0918) ccw
  arc A406 (42.1129, 1.2009) -> (42.4802, 1.0875) centre (43.1158, 3.7957) ccw
  arc A407 (41.5322, 1.4716) -> (42.1129, 1.2009) centre (43.7646, 5.5025) ccw
  arc A408 (40.8422, 1.9124) -> (41.5322, 1.4716) centre (44.6468, 7.1085) ccw
  arc A409 (41.7447, 2.8456) -> (40.9537, 2.6339) centre (43.011, -3.4687) ccw
  arc A410 (42.38, 2.9283) -> (41.7447, 2.8456) centre (42.6551, -1.6713) ccw
  arc A411 (42.7644, 2.9255) -> (42.38, 2.9283) centre (42.5522, 0.1517) ccw
  arc A412 (42.8546, 2.9152) -> (42.7644, 2.9255) centre (42.6929, 1.8946) ccw
  arc A413 (42.8546, 2.9152) -> (43.4106, 3.3149) centre (42.8984, 3.4409) ccw
  line L56 (43.4106, 3.3149) -> (43.4092, 3.3153)
  arc A414 (43.4092, 3.3153) -> (43.4138, 3.3287) centre (42.9126, 3.493) ccw
  arc A415 (43.4138, 3.3287) -> (43.4166, 3.3425) centre (42.8984, 3.4409) ccw
  line L57 (43.4166, 3.3425) -> (43.418, 3.3421)
  arc A416 (43.418, 3.3421) -> (43.1411, 3.9684) centre (42.9126, 3.493) ccw
  arc A417 (43.0582, 4.0053) -> (43.1411, 3.9684) centre (43.5188, 4.9303) ccw
  arc A418 (42.7254, 4.1976) -> (43.0582, 4.0053) centre (44.2805, 6.5042) ccw
  arc A419 (42.2195, 4.5908) -> (42.7254, 4.1976) centre (45.2928, 8.0238) ccw
  arc A420 (41.6448, 5.174) -> (42.2195, 4.5908) centre (46.5103, 9.3932) ccw
  arc A421 (42.7324, 5.883) -> (41.9142, 5.8526) centre (42.5619, -0.5548) ccw
  arc A422 (43.3702, 5.8222) -> (42.7324, 5.883) centre (42.6149, 1.2768) ccw
  arc A423 (43.7443, 5.734) -> (43.3702, 5.8222) centre (42.9202, 3.077) ccw
  arc A424 (43.8299, 5.7039) -> (43.7443, 5.734) centre (43.4452, 4.7449) ccw
  arc A425 (43.8299, 5.7039) -> (44.461, 5.9699) centre (43.9896, 6.2067) ccw
  line L58 (44.461, 5.9699) -> (44.4597, 5.9705)
  arc A426 (44.4597, 5.9705) -> (44.4671, 5.9825) centre (44.015, 6.2543) ccw
  arc A427 (44.4671, 5.9825) -> (44.473, 5.9954) centre (43.9896, 6.2067) ccw
  line L59 (44.473, 5.9954) -> (44.4742, 5.9947)
  arc A428 (44.4742, 5.9947) -> (44.3437, 6.6669) centre (44.015, 6.2543) ccw
  arc A429 (44.271, 6.7213) -> (44.3437, 6.6669) centre (44.9259, 7.5206) ccw
  arc A430 (43.9893, 6.9829) -> (44.271, 6.7213) centre (46.0188, 8.8856) ccw
  arc A431 (43.5836, 7.4787) -> (43.9893, 6.9829) centre (47.3438, 10.1418) ccw
  arc A432 (43.1531, 8.1752) -> (43.5836, 7.4787) centre (48.8355, 11.206) ccw
  arc A433 (44.3712, 8.6245) -> (43.5667, 8.7769) centre (42.7724, 2.386) ccw
  arc A434 (44.9795, 8.4233) -> (44.3712, 8.6245) centre (43.2317, 4.1599) ccw
  arc A435 (45.3246, 8.254) -> (44.9795, 8.4233) centre (43.9299, 5.847) ccw
  arc A436 (45.4014, 8.2056) -> (45.3246, 8.254) centre (44.8129, 7.3562) ccw
  arc A437 (45.4014, 8.2056) -> (46.0758, 8.3245) centre (45.6689, 8.6602) ccw
  line L60 (46.0758, 8.3245) -> (46.0747, 8.3254)
  arc A438 (46.0747, 8.3254) -> (46.0846, 8.3355) centre (45.7043, 8.701) ccw
  arc A439 (46.0846, 8.3355) -> (46.0932, 8.3467) centre (45.6689, 8.6602) ccw
  line L61 (46.0932, 8.3467) -> (46.0942, 8.3458)
  arc A440 (46.0942, 8.3458) -> (46.1165, 9.0302) centre (45.7043, 8.701) ccw
  arc A441 (46.0578, 9.0994) -> (46.1165, 9.0302) centre (46.8741, 9.7329) ccw
  arc A442 (45.8414, 9.4171) -> (46.0578, 9.0994) centre (48.2433, 10.8205) ccw
  arc A443 (45.5562, 9.9908) -> (45.8414, 9.4171) centre (49.8147, 11.7504) ccw
  arc A444 (45.2915, 10.7656) -> (45.5562, 9.9908) centre (51.5058, 12.4559) ccw
  arc A445 (46.579, 10.9325) -> (45.8286, 11.2602) centre (43.6321, 5.2062) ccw
  arc A446 (47.1272, 10.601) -> (46.579, 10.9325) centre (44.4745, 6.8334) ccw
  arc A447 (47.426, 10.3592) -> (47.1272, 10.601) centre (45.5307, 8.3229) ccw
  arc A448 (47.4901, 10.2949) -> (47.426, 10.3592) centre (46.7274, 9.5978) ccw
  arc A449 (47.4901, 10.2949) -> (48.1741, 10.2608) centre (47.8521, 10.6786) ccw
  line L62 (48.1741, 10.2608) -> (48.1732, 10.2619)
  arc A450 (48.1732, 10.2619) -> (48.1851, 10.2695) centre (47.8957, 10.7105) ccw
  arc A451 (48.1851, 10.2695) -> (48.1959, 10.2786) centre (47.8521, 10.6786) ccw
  line L63 (48.1959, 10.2786) -> (48.1968, 10.2774)
  arc A452 (48.1968, 10.2774) -> (48.3708, 10.9397) centre (47.8957, 10.7105) ccw
  arc A453 (48.3289, 11.0202) -> (48.3708, 10.9397) centre (49.2658, 11.4562) ccw
  arc A454 (48.1887, 11.3781) -> (48.3289, 11.0202) centre (50.8426, 12.2119) ccw
  arc A455 (48.0382, 12.0009) -> (48.1887, 11.3781) centre (52.5815, 12.7687) ccw
  arc A456 (47.9526, 12.8152) -> (48.0382, 12.0009) centre (54.3872, 13.0803) ccw
  arc A457 (49.245, 12.6914) -> (48.5863, 13.1778) centre (45.0977, 7.7644) ccw
  arc A458 (49.7057, 12.2462) -> (49.245, 12.6914) centre (46.2812, 9.1634) ccw
  arc A459 (49.9432, 11.944) -> (49.7057, 12.2462) centre (47.6423, 10.3805) ccw
  arc A460 (49.9914, 11.8671) -> (49.9432, 11.944) centre (49.0926, 11.3571) ccw
  arc A461 (49.9914, 11.8671) -> (50.6506, 11.6816) centre (50.4297, 12.1606) ccw
  line L64 (50.6506, 11.6816) -> (50.65, 11.6829)
  arc A462 (50.65, 11.6829) -> (50.6633, 11.6876) centre (50.4793, 12.182) ccw
  arc A463 (50.6633, 11.6876) -> (50.6759, 11.6941) centre (50.4297, 12.1606) ccw
  line L65 (50.6759, 11.6941) -> (50.6764, 11.6927)
  arc A464 (50.6764, 11.6927) -> (50.9935, 12.2997) centre (50.4793, 12.182) ccw
  arc A465 (50.9706, 12.3875) -> (50.9935, 12.2997) centre (51.981, 12.6041) ccw
  arc A466 (50.9135, 12.7677) -> (50.9706, 12.3875) centre (53.6864, 12.9899) ccw
  arc A467 (50.9054, 13.4083) -> (50.9135, 12.7677) centre (55.5056, 13.1459) ccw
  arc A468 (51.0031, 14.2212) -> (50.9054, 13.4083) centre (57.3354, 13.0478) ccw
  arc A469 (52.2355, 13.813) -> (51.7016, 14.4338) centre (47.0959, 9.9324) ccw
  arc A470 (52.5856, 13.2765) -> (52.2355, 13.813) centre (48.561, 11.0329) ccw
  arc A471 (52.7499, 12.9289) -> (52.5856, 13.2765) centre (50.1588, 11.9166) ccw
  arc A472 (52.7798, 12.8432) -> (52.7499, 12.9289) centre (51.7901, 12.5461) ccw
  arc A473 (52.7798, 12.8432) -> (53.3812, 12.5157) centre (53.2724, 13.0318) ccw
  line L66 (53.3812, 12.5157) -> (53.3809, 12.5171)
  arc A474 (53.3809, 12.5171) -> (53.3949, 12.5188) centre (53.3255, 13.0417) ccw
  arc A475 (53.3949, 12.5188) -> (53.4086, 12.5222) centre (53.2724, 13.0318) ccw
  line L67 (53.4086, 12.5222) -> (53.4089, 12.5208)
  arc A476 (53.4089, 12.5208) -> (53.853, 13.042) centre (53.3255, 13.0417) ccw
  arc A477 (53.8502, 13.1327) -> (53.853, 13.042) centre (54.8835, 13.1191) ccw
  arc A478 (53.8791, 13.5161) -> (53.8502, 13.1327) centre (56.632, 13.1157) ccw
  arc A479 (54.0138, 14.1424) -> (53.8791, 13.5161) centre (58.4404, 12.863) ccw
  arc A480 (54.29, 14.9132) -> (54.0138, 14.1424) centre (60.2024, 12.3602) ccw
  arc A481 (55.4007, 14.241) -> (55.0183, 14.965) centre (49.5264, 11.6013) ccw
  arc A482 (55.6226, 13.64) -> (55.4007, 14.241) centre (51.1996, 12.3483) ccw
  arc A483 (55.7054, 13.2646) -> (55.6226, 13.64) centre (52.954, 12.8543) ccw
  arc A484 (55.7155, 13.1744) -> (55.7054, 13.2646) centre (54.6845, 13.1049) ccw
  arc A485 (55.7155, 13.1744) -> (56.2289, 12.7213) centre (56.2377, 13.2487) ccw
  line L68 (56.2289, 12.7213) -> (56.229, 12.7227)
  arc A486 (56.229, 12.7227) -> (56.243, 12.7212) centre (56.2917, 13.2465) ccw
  arc A487 (56.243, 12.7212) -> (56.2571, 12.7215) centre (56.2377, 13.2487) ccw
  line L69 (56.2571, 12.7215) -> (56.257, 12.7201)
  arc A488 (56.257, 12.7201) -> (56.806, 13.1294) centre (56.2917, 13.2465) ccw
  arc A489 (56.8235, 13.2185) -> (56.806, 13.1294) centre (57.8278, 12.9752) ccw
  arc A490 (56.937, 13.5858) -> (56.8235, 13.2185) centre (59.5318, 12.5828) ccw
  arc A491 (57.2077, 14.1664) -> (56.937, 13.5858) centre (61.2385, 11.9341) ccw
  arc A492 (57.6484, 14.8565) -> (57.2077, 14.1664) centre (62.8445, 11.0518) ccw
  arc A493 (0.5315, 8.0348) -> (-0.1111, 7.9527) centre (1.2232, 0.0647) ccw
  arc A494 (-2.858, 6.9454) -> (-3.4014, 6.5926) centre (1.2232, 0.0647) ccw
  arc A495 (-5.4393, 4.4932) -> (-5.7758, 3.9396) centre (1.2232, 0.0647) ccw
  arc A496 (-6.701, 1.1639) -> (-6.7639, 0.5192) centre (1.2232, 0.0647) ccw
  arc A497 (-6.3932, -2.3831) -> (-6.1701, -2.9913) centre (1.2232, 0.0647) ccw
  arc A498 (-4.5769, -5.4453) -> (-4.112, -5.8965) centre (1.2232, 0.0647) ccw
  arc A499 (-1.6118, -7.4161) -> (-0.9972, -7.621) centre (1.2232, 0.0647) ccw
  arc A500 (1.9148, -7.9053) -> (2.5574, -7.8232) centre (1.2232, 0.0647) ccw
  arc A501 (5.3044, -6.816) -> (5.8477, -6.4632) centre (1.2232, 0.0647) ccw
  arc A502 (7.8856, -4.3638) -> (8.2221, -3.8102) centre (1.2232, 0.0647) ccw
  arc A503 (9.1473, -1.0345) -> (9.2102, -0.3897) centre (1.2232, 0.0647) ccw
  arc A504 (8.8395, 2.5125) -> (8.6164, 3.1207) centre (1.2232, 0.0647) ccw
  arc A505 (7.0232, 5.5747) -> (6.5583, 6.0259) centre (1.2232, 0.0647) ccw
  arc A506 (4.0581, 7.5456) -> (3.4435, 7.7504) centre (1.2232, 0.0647) ccw
  arc A507 (44.4385, -9.9074) -> (44.933, -10.4446) centre (55.7173, -0.0187) ccw
  arc A508 (46.9217, -12.1693) -> (47.5234, -12.5829) centre (55.7173, -0.0187) ccw
  arc A509 (49.846, -13.8219) -> (50.5246, -14.0912) centre (55.7173, -0.0187) ccw
  arc A510 (53.0647, -14.7823) -> (53.7863, -14.8939) centre (55.7173, -0.0187) ccw
  arc A511 (56.4164, -15.0024) -> (57.1447, -14.9506) centre (55.7173, -0.0187) ccw
  arc A512 (59.7331, -14.4712) -> (60.4316, -14.2586) centre (55.7173, -0.0187) ccw
  arc A513 (62.8484, -13.2152) -> (63.4821, -12.8526) centre (55.7173, -0.0187) ccw
  arc A514 (65.6061, -11.2976) -> (66.1432, -10.803) centre (55.7173, -0.0187) ccw
  arc A515 (67.8679, -8.8143) -> (68.2815, -8.2126) centre (55.7173, -0.0187) ccw
  arc A516 (69.5205, -5.89) -> (69.7899, -5.2114) centre (55.7173, -0.0187) ccw
  arc A517 (70.4809, -2.6713) -> (70.5925, -1.9498) centre (55.7173, -0.0187) ccw
  arc A518 (70.701, 0.6804) -> (70.6493, 1.4087) centre (55.7173, -0.0187) ccw
  arc A519 (70.1698, 3.997) -> (69.9573, 4.6956) centre (55.7173, -0.0187) ccw
  arc A520 (68.9139, 7.1123) -> (68.5512, 7.746) centre (55.7173, -0.0187) ccw
  arc A521 (66.9962, 9.87) -> (66.5016, 10.4072) centre (55.7173, -0.0187) ccw
  arc A522 (64.513, 12.1319) -> (63.9113, 12.5455) centre (55.7173, -0.0187) ccw
  arc A523 (61.5887, 13.7845) -> (60.91, 14.0538) centre (55.7173, -0.0187) ccw
  arc A524 (58.37, 14.7449) -> (57.6484, 14.8565) centre (55.7173, -0.0187) ccw
  arc A525 (55.0183, 14.965) -> (54.29, 14.9132) centre (55.7173, -0.0187) ccw
  arc A526 (51.7016, 14.4338) -> (51.0031, 14.2212) centre (55.7173, -0.0187) ccw
  arc A527 (48.5863, 13.1778) -> (47.9526, 12.8152) centre (55.7173, -0.0187) ccw
  arc A528 (45.8286, 11.2602) -> (45.2915, 10.7656) centre (55.7173, -0.0187) ccw
  arc A529 (43.5667, 8.7769) -> (43.1531, 8.1752) centre (55.7173, -0.0187) ccw
  arc A530 (41.9142, 5.8526) -> (41.6448, 5.174) centre (55.7173, -0.0187) ccw
  arc A531 (40.9537, 2.6339) -> (40.8422, 1.9124) centre (55.7173, -0.0187) ccw
  arc A532 (40.7336, -0.7178) -> (40.7854, -1.4461) centre (55.7173, -0.0187) ccw
  arc A533 (41.2649, -4.0344) -> (41.4774, -4.733) centre (55.7173, -0.0187) ccw
  arc A534 (42.5208, -7.1497) -> (42.8834, -7.7834) centre (55.7173, -0.0187) ccw
  line L70 (-23.2216, 0.0536) -> (50.2634, 0.0536)
  point P0 (-6.701, 1.1639)
  point P1 (-6.7521, 0.6928)
  point P2 (-6.3932, -2.3831)
  point P3 (-6.1701, -2.9913)
  point P4 (-4.5769, -5.4453)
  point P5 (-4.112, -5.8965)
  point P6 (-1.6118, -7.4161)
  point P7 (-0.9972, -7.621)
  point P8 (1.9148, -7.9053)
  point P9 (2.5574, -7.8232)
  point P10 (5.3044, -6.816)
  point P11 (5.8477, -6.4632)
  point P12 (7.8856, -4.3638)
  point P13 (8.2221, -3.8102)
  point P14 (9.1473, -1.0345)
  point P15 (9.2102, -0.3897)
  point P16 (8.8395, 2.5125)
  point P17 (8.6164, 3.1207)
  point P18 (7.0232, 5.5747)
  point P19 (6.5583, 6.0259)
  point P20 (4.0581, 7.5456)
  point P21 (3.4435, 7.7504)
  point P22 (0.5315, 8.0348)
  point P23 (-0.1111, 7.9527)
  point P24 (-2.858, 6.9454)
  point P25 (-3.4014, 6.5926)
  point P26 (-5.4393, 4.4932)
  point P27 (-5.7758, 3.9396)
  point P28 (58.37, 14.7449)
  point P29 (57.6484, 14.8565)
  point P30 (55.0183, 14.965)
  point P31 (54.29, 14.9132)
  point P32 (51.7016, 14.4338)
  point P33 (51.0031, 14.2212)
  point P34 (48.5863, 13.1778)
  point P35 (47.9526, 12.8152)
  point P36 (45.8286, 11.2602)
  point P37 (45.2915, 10.7656)
  point P38 (43.5667, 8.7769)
  point P39 (43.1531, 8.1752)
  point P40 (41.9142, 5.8526)
  point P41 (41.6448, 5.174)
  point P42 (40.9537, 2.6339)
  point P43 (40.8422, 1.9124)
  point P44 (40.7336, -0.7178)
  point P45 (40.7854, -1.4461)
  point P46 (41.2649, -4.0344)
  point P47 (41.4774, -4.733)
  point P48 (42.5208, -7.1497)
  point P49 (42.8834, -7.7834)
  point P50 (44.4385, -9.9074)
  point P51 (44.933, -10.4446)
  point P52 (46.9217, -12.1693)
  point P53 (47.5234, -12.5829)
  point P54 (49.846, -13.8219)
  point P55 (50.5246, -14.0912)
  point P56 (53.0647, -14.7823)
  point P57 (53.7863, -14.8939)
  point P58 (56.4164, -15.0024)
  point P59 (57.1447, -14.9506)
  point P60 (59.7331, -14.4712)
  point P61 (60.4316, -14.2586)
  point P62 (62.8484, -13.2152)
  point P63 (63.4821, -12.8526)
  point P64 (65.6061, -11.2976)
  point P65 (66.1432, -10.803)
  point P66 (67.8679, -8.8143)
  point P67 (68.2815, -8.2126)
  point P68 (69.5205, -5.89)
  point P69 (69.7899, -5.2114)
  point P70 (70.4809, -2.6713)
  point P71 (70.5925, -1.9498)
  point P72 (70.701, 0.6804)
  point P73 (70.6493, 1.4087)
  point P74 (70.1698, 3.997)
  point P75 (69.9573, 4.6956)
  point P76 (68.9139, 7.1123)
  point P77 (68.5512, 7.746)
  point P78 (66.9962, 9.87)
  point P79 (66.5016, 10.4072)
  point P80 (64.513, 12.1319)
  point P81 (63.9113, 12.5455)
  point P82 (61.5887, 13.7845)
  point P83 (60.91, 14.0538)
  constraints: 1010 point on circle, 507 centre point, 142 end point, 1 horizontal, 84 other